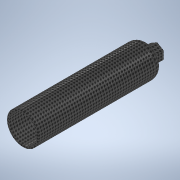
# Autodesk Inventor part: pegsFront wheel
Saved by Autodesk Inventor 2022.2 (Build 262287010, 287A)
## iProperties
Created: 2022-04-06
Part Number: pegsFront wheel
Material: Steel, Alloy
Document SubType Name: Modeling
Designer: Finn Oriwohl
Density: 7.73 g/cm^3
Appearance: Skid Plate
Author: Finn Oriwohl
Autodesk Inventor part; units mm, degrees
ref_plane "YZ Plane" through (0, 0, 0) normal (1, 0, 0) x (0, 1, 0)
ref_plane "XZ Plane" through (0, 0, 0) normal (0, 1, 0) x (-1, 0, 0)
ref_plane "XY Plane" through (0, 0, 0) normal (0, 0, 1) x (1, 0, 0)
sketch "Sketch1" plane through (0, 0, 0) normal (0, 0, 1) x (1, 0, 0)
  circle A0 centre (0, 0) radius 16.5
  circle A1 centre (0, 0) radius 14.5
  line L0 (7, -4.0415) -> (0, -8.0829)
  line L1 (0, -8.0829) -> (-7, -4.0415)
  line L2 (-7, -4.0415) -> (-7, 4.0415)
  line L3 (-7, 4.0415) -> (0, 8.0829)
  line L4 (0, 8.0829) -> (7, 4.0415)
  line L5 (7, 4.0415) -> (7, -4.0415)
  circle A2 centre (0, 0) radius 5
  dimension "d0" = 33
  dimension "d1" = 2
  dimension "d2" = 14
  dimension "d3" = 10
  constraints: 12 end point, 3 centre point, 3 coincident, 13 other
  measures "d0" diameter of A0
  measures "d1" radial gap between concentric circles of A0 A1
  measures "d2" distance between parallel lines of L5 L2
  measures "d3" diameter of A2
extrude "Extrusion1" add sketch "Sketch1" against normal blind 10 contours L0 L1 L2 L3 L4 L5
extrude "lenght'" add sketch "Sketch1" along normal blind 70 contours A0
extrude "Extrusion3" add sketch "Sketch1" along normal blind 3 contours A1
fillet "Fillet1" radius 7.75 1 edges at (-16.5, 0, 0)
thread "Thread1" size "M10x1.5" class "6H" standard "ANSI Metric M Profile" length 48
body "Solid1"
